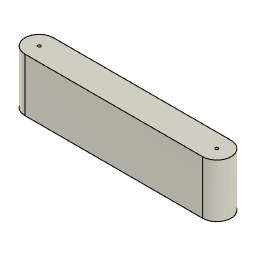
Robot Final attemp v10 (Autodesk Fusion 360 archive; units mm, degrees)
design "link1"
Autodesk Fusion 360 part; units mm, degrees
sketch "Boceto1" plane through (0, 0, 0) normal (0, 0, 1) x (1, 0, 0)
  line L0 (-65, 45) -> (185, 45)
  line L1 (185, 5) -> (-65, 5)
  arc A0 (185, 5) -> (185, 45) centre (185, 25) ccw
  arc A1 (-65, 45) -> (-65, 5) centre (-65, 25) ccw
  dimension "d3" = 40
  dimension "d4" = 40
  constraint horizontal L0
  constraint horizontal L1
  constraint tangent L1 A1
  measures "d3" diameter of A1
  measures "d4" diameter of A0
extrude "Extruir1" add sketch "Boceto1" along normal blind 75
sketch "Boceto2" plane through (0, 0, 75) normal (0, 0, 1) x (-1, 0, 0)
  arc A0 (-185, -5) -> (-185, -45) centre (-185, -25) ccw
  line L0 (-185, -45) -> (65, -45)
  arc A1 (65, -45) -> (65, -5) centre (65, -25) ccw
  line L1 (65, -5) -> (-185, -5)
  circle A2 centre (65, -25) radius 2
  circle A3 centre (-185, -25) radius 2
  dimension "d7" = 4
  dimension "d8" = 4
  constraint concentric A1 A2
  constraint concentric A0 A3
  measures "d7" diameter of A2
  measures "d8" diameter of A3
extrude "Extruir2" cut sketch "Boceto2" against normal blind 100 contours A2 | A3

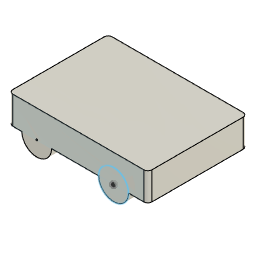
design "robot"
Autodesk Fusion 360 part; units mm, degrees
sketch "Boceto1" plane through (0, 0, 0) normal (0, 0, 1) x (1, 0, 0)
  line L0 (-168.6066, 213.4571) -> (161.3934, 213.4571)
  line L1 (171.3934, 203.4571) -> (171.3934, -26.5429)
  line L2 (161.3934, -36.5429) -> (-168.6066, -36.5429)
  line L3 (-178.6066, -26.5429) -> (-178.6066, 203.4571)
  arc A0 (-168.6066, 213.4571) -> (-178.6066, 203.4571) centre (-168.6066, 203.4571) ccw
  arc A1 (-178.6066, -26.5429) -> (-168.6066, -36.5429) centre (-168.6066, -26.5429) ccw
  arc A2 (171.3934, 203.4571) -> (161.3934, 213.4571) centre (161.3934, 203.4571) ccw
  arc A3 (161.3934, -36.5429) -> (171.3934, -26.5429) centre (161.3934, -26.5429) ccw
  point P0 (-178.6066, 213.4571)
  point P1 (171.3934, 213.4571)
  point P2 (-178.6066, -36.5429)
  dimension "d1" = 350
  dimension "d2" = 250
  dimension "d3" = 10
  dimension "d4" = 10
  dimension "d5" = 10
  dimension "d6" = 10
  constraint horizontal L0
  constraint vertical L1
  constraint horizontal L2
  constraint vertical L3
  constraint coincident P0 L3
  constraint coincident P0 L0
  constraint tangent L3 A0
  constraint tangent L0 A0
  constraint coincident P2 L3
  constraint coincident P2 L2
  constraint tangent L3 A1
  constraint tangent L2 A1
  constraint coincident P1 L0
  constraint coincident P1 L1
  constraint tangent L0 A2
  constraint tangent L1 A2
  constraint tangent L2 A3
  constraint tangent L1 A3
  measures "d1" distance of P0 P1
  measures "d2" distance of P0 P2
  measures "d3" radius of A0
  measures "d4" radius of A1
  measures "d5" radius of A2
  measures "d6" radius of A3
extrude "Extruir1" add sketch "Boceto1" along normal blind 70
sketch "Boceto2" plane through (0, -36.5429, 0) normal (0, -1, 0) x (1, 0, 0)
  line L0 (-168.6066, 0) -> (161.3934, 0)
  line L1 (161.3934, 0) -> (161.3934, 70)
  line L2 (161.3934, 70) -> (-168.6066, 70)
  line L3 (-168.6066, 70) -> (-168.6066, 0)
  circle A0 centre (85.2742, 0) radius 37.5
  dimension "d9" = 75
  constraint coincident L0 A0.centre
  measures "d9" diameter of A0
extrude "Extruir2" add sketch "Boceto2" against normal blind 250 contours L0 A0 picked at (94.9927, -12.1866)
sketch "Boceto3" plane through (0, -36.5429, 0) normal (0, -1, 0) x (1, 0, 0)
  circle A0 centre (-108.4383, 0.5063) radius 37.5
  dimension "d12" = 75
  measures "d12" diameter of A0
extrude "Extruir3" add sketch "Boceto3" against normal blind 250
sketch "Boceto4" plane through (0, 213.4571, 0) normal (0, 1, 0) x (-1, 0, 0)
  line L0 (145.9349, 0) -> (168.6066, 0)
  line L1 (168.6066, 0) -> (168.6066, 70)
  line L2 (168.6066, 70) -> (-161.3934, 70)
  line L3 (-161.3934, 70) -> (-161.3934, 0)
  line L4 (-161.3934, 0) -> (-122.7742, 0)
  arc A0 (-122.7742, 0) -> (-47.7742, 0) centre (-85.2742, 0) ccw
  line L5 (-47.7742, 0) -> (70.9417, 0)
  arc A1 (70.9417, 0) -> (145.9349, 0) centre (108.4383, 0.5063) ccw
  circle A2 centre (-85.2742, 0) radius 2
  circle A3 centre (108.4383, 0.5063) radius 2
  dimension "d15" = 4
  dimension "d16" = 4
  constraint concentric A0 A2
  constraint concentric A1 A3
  measures "d15" diameter of A2
  measures "d16" diameter of A3
extrude "Extruir4" cut sketch "Boceto4" against normal blind 300 contours A2 | A3

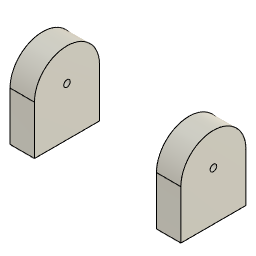
design "joint base-link1"
Autodesk Fusion 360 part; units mm, degrees
sketch "Boceto1" plane through (0, 0, 0) normal (0, 0, 1) x (1, 0, 0)
  line L0 (-50, 40) -> (25, 40)
  line L1 (25, 40) -> (25, 0)
  line L2 (25, 0) -> (-50, 0)
  line L3 (-50, 0) -> (-50, 40)
  line L4 (-50, 40) -> (-65, 40)
  line L5 (-65, 40) -> (-65, 0)
  line L6 (-65, 0) -> (-50, 0)
  line L7 (-50, 0) -> (-50, 40)
  line L8 (25, 40) -> (40, 40)
  line L9 (40, 40) -> (40, 0)
  line L10 (40, 0) -> (25, 0)
  line L11 (25, 0) -> (25, 40)
  dimension "d1" = 75
  dimension "d2" = 40
  dimension "d3" = 15
  dimension "d4" = 15
  constraint horizontal L0
  constraint vertical L1
  constraint horizontal L2
  constraint vertical L3
  constraint horizontal L4
  constraint vertical L5
  constraint horizontal L6
  constraint vertical L7
  constraint horizontal L8
  constraint vertical L9
  constraint horizontal L10
  constraint vertical L11
  measures "d1" distance of L0.start L0.end
  measures "d2" distance of L0.start L2.end
  measures "d3" distance of L0.start L4.end
  measures "d4" distance of L0.end L8.end
extrude "Extruir1" add sketch "Boceto1" along normal blind 50 contours L3 L4 L5 L6 L7 | L1 L8 L9 L10 L11 makes body 1 at (-50, 13.3333, 16.6667) makes body 2 at (40, 26.6667, 16.6667)
sketch "Boceto2" plane through (40, 0, 0) normal (1, 0, 0) x (0, 1, 0)
  line L0 (0, 0) -> (40, 0)
  line L1 (40, 0) -> (40, 50)
  line L2 (40, 50) -> (0, 50)
  line L3 (0, 50) -> (0, 0)
  circle A0 centre (20, 30) radius 20
  dimension "d7" = 40
  constraint tangent L2 A0
  constraint tangent L1 A0
  measures "d7" diameter of A0
extrude "Extruir2" cut sketch "Boceto2" against normal blind 115 contours L2 L3 A0 | L1 L2 A0 bodies 1 2
sketch "Boceto3" plane through (40, 0, 0) normal (1, 0, 0) x (0, 1, 0)
  arc A0 (40, 30) -> (0, 30) centre (20, 30) ccw
  line L0 (0, 30) -> (0, 0)
  line L1 (0, 0) -> (40, 0)
  line L2 (40, 0) -> (40, 30)
  circle A1 centre (20, 30) radius 2
  dimension "d10" = 4
  constraint concentric A0 A1
  measures "d10" diameter of A1
extrude "Extruir3" cut sketch "Boceto3" against normal blind 140 contours A1 bodies 1 2

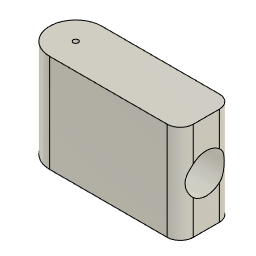
design "link3"
Autodesk Fusion 360 part; units mm, degrees
sketch "Boceto1" plane through (0, 0, 0) normal (0, 0, 1) x (1, 0, 0)
  line L0 (-36.4214, 37.7542) -> (19.5786, 37.7542)
  line L1 (19.5786, -2.2458) -> (-36.4214, -2.2458)
  arc A0 (-36.4214, 37.7542) -> (-36.4214, -2.2458) centre (-36.4214, 17.7542) ccw
  line L2 (-6.4214, 37.7542) -> (53.5786, 37.7542)
  line L3 (63.5786, 27.7542) -> (63.5786, 7.7542)
  line L4 (53.5786, -2.2458) -> (-6.4214, -2.2458)
  arc A1 (63.5786, 27.7542) -> (53.5786, 37.7542) centre (53.5786, 27.7542) ccw
  arc A2 (53.5786, -2.2458) -> (63.5786, 7.7542) centre (53.5786, 7.7542) ccw
  point P0 (63.5786, 37.7542)
  dimension "d3" = 40
  dimension "d11" = 70
  dimension "d12" = 40
  dimension "d14" = 10
  dimension "d15" = 10
  constraint horizontal L0
  constraint horizontal L1
  constraint tangent L0 A0
  constraint horizontal L2
  constraint vertical L3
  constraint horizontal L4
  constraint coincident L0 L2.start
  constraint coincident P0 L3
  constraint coincident P0 L2
  constraint tangent L3 A1
  constraint tangent L2 A1
  constraint tangent L3 A2
  constraint tangent L4 A2
  measures "d3" diameter of A0
  measures "d11" distance of L2.start P0
  measures "d12" distance of L2.start L4.end
  measures "d14" radius of A1
  measures "d15" radius of A2
extrude "Extruir1" add sketch "Boceto1" along normal blind 75
sketch "Boceto2" plane through (0, 0, 75) normal (0, 0, 1) x (-1, 0, 0)
  arc A0 (36.4214, -37.7542) -> (36.4214, 2.2458) centre (36.4214, -17.7542) ccw
  line L0 (36.4214, 2.2458) -> (-53.5786, 2.2458)
  line L1 (-53.5786, -37.7542) -> (36.4214, -37.7542)
  circle A1 centre (36.4214, -17.7542) radius 2
  arc A2 (-53.5786, 2.2458) -> (-63.5786, -7.7542) centre (-53.5786, -7.7542) ccw
  line L2 (-63.5786, -7.7542) -> (-63.5786, -27.7542)
  arc A3 (-63.5786, -27.7542) -> (-53.5786, -37.7542) centre (-53.5786, -27.7542) ccw
  dimension "d8" = 4
  constraint concentric A0 A1
  measures "d8" diameter of A1
extrude "Extruir2" cut sketch "Boceto2" against normal blind 110 contours A1
sketch "Boceto3" plane through (63.5786, 0, 0) normal (1, 0, 0) x (0, 1, 0)
  line L0 (7.7542, 0) -> (27.7542, 0)
  line L1 (27.7542, 0) -> (27.7542, 75)
  line L2 (27.7542, 75) -> (7.7542, 75)
  line L3 (7.7542, 75) -> (7.7542, 0)
  circle A0 centre (17.7542, 37.5) radius 15
  line L4 (-2.2458, 0) -> (-2.2458, 75)
  dimension "d16" = 30
  dimension "d17" = 37.5
  dimension "d18" = 20
  measures "d16" diameter of A0
  measures "d17" distance of L2 A0.centre
  measures "d18" distance of A0.centre L4
extrude "Extruir3" cut sketch "Boceto3" against normal blind 70 contours L3 A0 | L1 L3 A0 | L1 A0

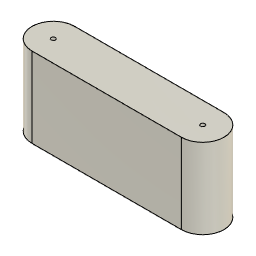
design "link2"
Autodesk Fusion 360 part; units mm, degrees
sketch "Boceto1" plane through (0, 0, 0) normal (0, 0, 1) x (1, 0, 0)
  line L0 (-60, 30) -> (80, 30)
  line L1 (80, -10) -> (-60, -10)
  arc A0 (80, -10) -> (80, 30) centre (80, 10) ccw
  arc A1 (-60, 30) -> (-60, -10) centre (-60, 10) ccw
  dimension "d3" = 40
  dimension "d4" = 40
  constraint horizontal L0
  constraint horizontal L1
  constraint tangent L0 A1
  measures "d3" diameter of A1
  measures "d4" diameter of A0
extrude "Extruir1" add sketch "Boceto1" along normal blind 75
sketch "Boceto2" plane through (0, 0, 0) normal (1, 0, 0) x (0, 1, 0)
sketch "Boceto3" plane through (0, 0, 75) normal (0, 0, 1) x (-1, 0, 0)
  arc A0 (-80, 10) -> (-80, -30) centre (-80, -10) ccw
  line L0 (-80, -30) -> (60, -30)
  arc A1 (60, -30) -> (60, 10) centre (60, -10) ccw
  line L1 (60, 10) -> (-80, 10)
  circle A2 centre (-80, -10) radius 2
  circle A3 centre (60, -10) radius 2
  dimension "d7" = 4
  dimension "d8" = 4
  constraint concentric A0 A2
  constraint concentric A1 A3
  measures "d7" diameter of A2
  measures "d8" diameter of A3
extrude "Extruir2" cut sketch "Boceto3" against normal blind 110 contours A2 | A3
